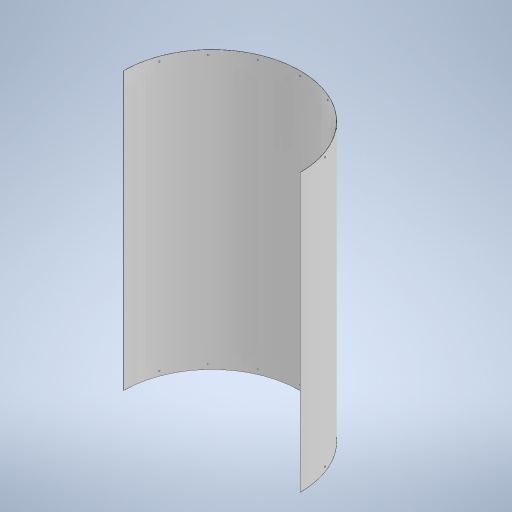
# Autodesk Inventor part: Aspa1
Saved by Autodesk Inventor 2024 (Build 280153000, 153)
## iProperties
Created: 2024-04-25
Part Number: Aspa1
Material: Genérico
Document SubType Name: Modeling
Designer: alexa
Density: 1 g/cm^3
Appearance: Valor por defecto
Author: alexa
Autodesk Inventor part; units mm, degrees
note: some values were not read from the file. Chosen so that the rebuilt part matches the saved one: pattern direction of "Circular Pattern2".
ref_plane "YZ Plane" through (0, 0, 0) normal (1, 0, 0) x (0, 1, 0)
sketch "Sketch2" plane through (0, 0, 0) normal (1, 0, 0) x (0, 1, 0)
  line L0 (0, 0) -> (121.8561, 0)
  line L1 (3, -194.17) -> (497, -194.17)
  line L2 (610, -194.17) -> (610, -194.44)
  line L3 (610, -194.44) -> (0, -194.44)
  line L4 (0, -194.44) -> (0, -194.17)
  line L5 (500, 0) -> (497, 0)
  line L6 (3, -194.17) -> (0, -194.17)
  line L7 (497, -194.17) -> (610, -194.17)
  point P0 (3, 0)
  dimension "d7" = 610
  dimension "d34" = 194.17
  dimension "d36" = 0.27
  constraints: 16 end point, 5 horizontal, 2 parallel, 1 perpendicular, 1 point on line
  measures "d7" distance of L2.end L3.end
  measures "d34" distance of L0.start L4.end
  measures "d36" distance between parallel lines of L3 L7
revolve "Revolution1" add sketch "Sketch2" angle 180 mid plane about axis through (0, 0, 0) along (0, 1, 0)
ref_plane "Work Plane2" through (0, 0, -197.17) normal (0, 0, 1) x (1, 0, 0)
sketch "Sketch5" plane through (0, 0, -197.17) normal (0, 0, 1) x (1, 0, 0)
  line L0 (194.17, 610) -> (-194.17, 610) projected
  circle A0 centre (0, 600) radius 1.5
  point P0 (0, 0)
  point P1 (0, 610)
  dimension "d24" = 3
  dimension "d35" = 10
  constraints: 1 centre point, 1 midpoint
  measures "d24" diameter of A0
  measures "d35" distance of point (0, 610) A0.centre
extrude "Extrusion3" cut sketch "Sketch5" along normal blind 5
ref_plane "Work Plane3" through (0, 305, 0) normal (0, 1, 0) x (1, 0, 0)
mirror "Mirror1" about plane through (0, 305, 0) normal (0, 1, 0) of "Extrusion3"
pattern_circular "Circular Pattern2" count 7 over 140 about axis through (0, -10, 0) along (0, 1, 0) of "Extrusion3", "Mirror1" both ways yes
body "Solid2"
